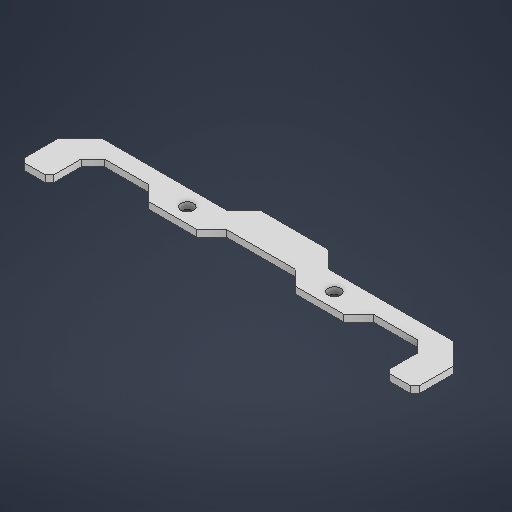
# Autodesk Inventor part: PCBDummy - SenRigFront
Saved by Autodesk Inventor 2027 (Build 310192000, 192)
## iProperties
Created: 2026-09-26
Part Number: PCBDummy - SenRigFront
Material: Všeobecné
Document SubType Name: Modeling
Designer: Vadim
Density: 1 g/cm^3
Appearance: Výchozí
Author: Vadim
Autodesk Inventor part; units mm, degrees
ref_plane "YZ Plane" through (0, 0, 0) normal (1, 0, 0) x (0, 1, 0)
ref_plane "XZ Plane" through (0, 0, 0) normal (0, 1, 0) x (-1, 0, 0)
ref_plane "XY Plane" through (0, 0, 0) normal (0, 0, 1) x (1, 0, 0)
sketch "Náčrt1" plane through (0, 0, 0) normal (0, 1, 0) x (-1, 0, 0)
  line L0 (0, 0) -> (0, -9)
  line L1 (39.5, 0) -> (39.5, 9.8)
  line L2 (39.5, 9.8) -> (47.5, 9.8)
  line L3 (47.5, 9.8) -> (47.5, 0)
  line L4 (47.5, 0) -> (42.5, -5)
  line L5 (42.5, -5) -> (12, -5)
  line L6 (39.5, 0) -> (26.5, 0)
  line L7 (26.5, 0) -> (23.5, 3)
  line L8 (23.5, 3) -> (11.5, 3)
  line L9 (11.5, 3) -> (8.5, 0)
  line L10 (8.5, 0) -> (0, 0)
  circle A0 centre (17.5, -1) radius 1.5
  line L11 (12, -5) -> (8, -9)
  line L12 (8, -9) -> (0, -9)
  line L13 (17.5, 3) -> (17.5, -5) construction
  line L14 (39.5, 2) -> (37.5, 0)
  line L15 (11.7071, 2.5) -> (23.2929, 2.5)
  line L16 (23.2929, 2.5) -> (26.2929, -0.5)
  line L17 (26.2929, -0.5) -> (40, -0.5)
  line L18 (40, -0.5) -> (40, 9.3)
  line L19 (40, 9.3) -> (47, 9.3)
  line L20 (47, 9.3) -> (47, 0.2071)
  line L21 (47, 0.2071) -> (42.2929, -4.5)
  line L22 (42.2929, -4.5) -> (11.7929, -4.5)
  line L23 (11.7929, -4.5) -> (7.7929, -8.5)
  line L24 (7.7929, -8.5) -> (0.5, -8.5)
  line L25 (0.5, -8.5) -> (0.5, -0.5)
  line L26 (0.5, -0.5) -> (8.7071, -0.5)
  line L27 (8.7071, -0.5) -> (11.7071, 2.5)
  line L28 (40, 1.7929) -> (37.7071, -0.5)
  line L29 (0.5, -0.5) -> (0, -0.5)
  line L30 (42.2929, -4.5) -> (41.7929, -5)
  line L31 (37.7071, -0.5) -> (37.2071, -1)
  line L32 (26.7929, -1) -> (26.2929, -0.5)
  line L33 (37.2071, -1) -> (26.7929, -1)
  line L34 (8.7071, -0.5) -> (8.2071, -1)
  line L35 (8.2071, -1) -> (0, -1)
  point P0 (17.5, -1)
  point P1 (38.5, 1)
  point P2 (47, -0.5)
  point P3 (38.2071, 0)
  point P4 (39.5, 1.2929)
  dimension "d1" = 4
  dimension "d2" = 4
  dimension "d3" = 3
  dimension "d4" = 6
  dimension "d5" = 8
  dimension "d6" = 2
  dimension "d7" = 2
  dimension "d8" = 3
  dimension "d9" = 17.5
  dimension "d10" = 5
  dimension "d11" = 5
  dimension "d12" = 14.8
  dimension "d13" = 22
  dimension "d14" = 8
  dimension "d15" = 4
  dimension "d16" = 45
  dimension "d24" = 0.5
  dimension "d25" = 0.5
  dimension "d27" = 0.5
  constraints: 74 end point, 12 perpendicular, 10 point on line, 6 collinear, 6 parallel, 4 midpoint, 2 vertical, 1 centre point, 1 horizontal, 13 other
  measures "d1" distance from line of L5 A0.centre
  measures "d2" distance from line of L8 A0.centre
  measures "d3" diameter of A0
  measures "d4" horizontal distance of A0.centre L7.end
  measures "d5" distance of L1.end L2.end
  measures "d6" distance of L1.start L14.end
  measures "d7" distance of L14.start L1.start
  measures "d8" horizontal distance of L7.end L6.end
  measures "d9" distance from line of L0 point (17.5, -1)
  measures "d10" horizontal distance of L3.end L4.end
  measures "d11" horizontal distance of L3.end L4.end
  measures "d12" distance between parallel lines of L2 L5
  measures "d13" distance from line of L1 point (17.5, -1)
  measures "d14" distance of L11.end L0.end
  measures "d15" distance between parallel lines of L12 L5
  measures "d16" angle of L5 L11
  measures "d24" distance between parallel lines of L6 L17
  measures "d25" distance from line of point (38.5, 1) L28
  measures "d27" distance between parallel lines of L33 L17
extrude "Vysunutí1" add sketch "Náčrt1" along normal blind 1.6 contours L35 L25 L24 L23 L22 L30 L5 L11 L12 L0 | L35 L34 L27 L15 L16 L32 L33 L31 L17 L18 L19 L20 L21 L22 L23 L24 L25 | L28 L1 L6 | L6 L1 L28 L18 L17
chamfer "Zkosení1" distance 1 angle 45 2 edges at (-40, 0.8, 9.3) (-47, 0.8, 9.3)
mirror "Zrcadlit1" about plane through (0, 0, -1) normal (1, 0, 0)
sketch "Náčrt2" plane through (0, 0, 0) normal (0, -1, 0) x (1, 0, 0)
  circle A0 centre (17.5, -1) radius 1.5 projected
  line L0 (-12, -5) -> (-41.7929, -5) projected
  line L1 (-8, -9) -> (-12, -5) projected
  line L2 (-8, -9) -> (8, -9) projected
  line L3 (8, -9) -> (12, -5) projected
  line L4 (12, -5) -> (41.7929, -5) projected
  circle A1 centre (-17.5, -1) radius 1.5 projected
  line L5 (0, -9) -> (0, 0) construction
  line L6 (12, -9) -> (-12, -9) construction
  line L7 (-12, -9) -> (-12, -1) construction
  line L8 (-12, -1) -> (12, -1) construction
  line L9 (12, -1) -> (12, -9) construction
  line L10 (-40, 1.7929) -> (-37.2071, -1) projected
  line L11 (40, 1.7929) -> (37.2071, -1) projected
  line L12 (-47, 8.3) -> (-46, 9.3) projected
  line L13 (-47, 0.2071) -> (-47, 8.3) projected
  line L14 (-41.7929, -5) -> (-47, 0.2071) projected
  line L15 (41.7929, -5) -> (47, 0.2071) projected
  line L16 (47, 0.2071) -> (47, 8.3) projected
  line L17 (47, 8.3) -> (46, 9.3) projected
  line L18 (46, 9.3) -> (41, 9.3) projected
  line L19 (41, 9.3) -> (40, 8.3) projected
  line L20 (40, 8.3) -> (40, 1.7929) projected
  line L21 (26.7929, -1) -> (23.2929, 2.5) projected
  line L22 (23.2929, 2.5) -> (11.7071, 2.5) projected
  line L23 (11.7071, 2.5) -> (8.2071, -1) projected
  line L24 (-11.7071, 2.5) -> (-8.2071, -1) projected
  line L25 (-23.2929, 2.5) -> (-11.7071, 2.5) projected
  line L26 (-26.7929, -1) -> (-23.2929, 2.5) projected
  line L27 (-40, 8.3) -> (-40, 1.7929) projected
  line L28 (-41, 9.3) -> (-40, 8.3) projected
  line L29 (-46, 9.3) -> (-41, 9.3) projected
  line L30 (37.2071, -1) -> (26.7929, -1) projected
  line L31 (-37.2071, -1) -> (-26.7929, -1) projected
  line L32 (-8.2071, -1) -> (8.2071, -1) projected
  spline S0 degree 2 poles (6.8074, -7.598) (6.8074, -7.4522) (6.9114, -7.1896) (7.0044, -7.0984) knots 0 0 0 1 2 2 2
  spline S1 degree 2 poles (7.0044, -7.0984) (7.121, -6.9836) (7.4365, -6.865) (7.6772, -6.865) knots 0 0 0 1 2 2 2
  line L33 (7.6772, -6.865) -> (7.9306, -6.865)
  line L34 (7.9306, -6.865) -> (7.9306, -6.0263)
  line L35 (7.9306, -6.0263) -> (8.2296, -6.0263)
  line L36 (8.2296, -6.0263) -> (8.2296, -8.2763)
  line L37 (8.2296, -8.2763) -> (7.6644, -8.2763)
  spline S2 degree 2 poles (7.6644, -8.2763) (7.4638, -8.2763) (7.183, -8.2107) (7.0755, -8.1359) knots 0 0 0 1 2 2 2
  spline S3 degree 2 poles (7.0755, -8.1359) (6.9497, -8.0502) (6.8074, -7.7858) (6.8074, -7.598) knots 0 0 0 1 2 2 2
  spline S4 degree 2 poles (7.1192, -7.5889) (7.1192, -7.7056) (7.1995, -7.877) (7.2815, -7.9317) knots 0 0 0 1 2 2 2
  spline S5 degree 2 poles (7.2815, -7.9317) (7.3526, -7.9791) (7.5422, -8.0174) (7.6826, -8.0174) knots 0 0 0 1 2 2 2
  line L38 (7.6826, -8.0174) -> (7.9306, -8.0174)
  line L39 (7.9306, -8.0174) -> (7.9306, -7.1203)
  line L40 (7.9306, -7.1203) -> (7.7264, -7.1203)
  spline S6 degree 2 poles (7.7264, -7.1203) (7.5441, -7.1203) (7.3198, -7.1787) (7.2469, -7.2552) knots 0 0 0 1 2 2 2
  spline S7 degree 2 poles (7.2469, -7.2552) (7.1794, -7.3227) (7.1192, -7.4813) (7.1192, -7.5889) knots 0 0 0 1 2 2 2
  spline S8 degree 2 poles (5.6441, -5.9862) (5.8629, -5.9862) (6.2331, -6.1339) (6.368, -6.2816) knots 0 0 0 1 2 2 2
  spline S9 degree 2 poles (6.368, -6.2816) (6.5029, -6.4274) (6.6506, -6.865) (6.6506, -7.1495) knots 0 0 0 1 2 2 2
  spline S10 degree 2 poles (6.6506, -7.1495) (6.6506, -7.4321) (6.5066, -7.8515) (6.3698, -8.0065) knots 0 0 0 1 2 2 2
  spline S11 degree 2 poles (6.3698, -8.0065) (6.2349, -8.1578) (5.8666, -8.3164) (5.6387, -8.3164) knots 0 0 0 1 2 2 2
  spline S12 degree 2 poles (5.6387, -8.3164) (5.5256, -8.3164) (5.3269, -8.2836) (5.243, -8.2581) knots 0 0 0 1 2 2 2
  spline S13 degree 2 poles (5.243, -8.2581) (5.1701, -8.2344) (5.0187, -8.1669) (4.944, -8.1268) knots 0 0 0 1 2 2 2
  line L41 (4.944, -8.1268) -> (4.944, -7.7658)
  line L42 (4.944, -7.7658) -> (4.9677, -7.7658)
  spline S14 degree 2 poles (4.9677, -7.7658) (5.0078, -7.8022) (5.1318, -7.9043) (5.2211, -7.9536) knots 0 0 0 1 2 2 2
  spline S15 degree 2 poles (5.2211, -7.9536) (5.3068, -8.001) (5.5092, -8.0612) (5.6405, -8.0612) knots 0 0 0 1 2 2 2
  spline S16 degree 2 poles (5.6405, -8.0612) (5.7845, -8.0612) (6.0416, -7.9426) (6.1383, -7.8296) knots 0 0 0 1 2 2 2
  spline S17 degree 2 poles (6.1383, -7.8296) (6.2331, -7.7147) (6.3388, -7.3665) (6.3388, -7.1495) knots 0 0 0 1 2 2 2
  spline S18 degree 2 poles (6.3388, -7.1495) (6.3388, -6.9179) (6.2276, -6.5843) (6.131, -6.4694) knots 0 0 0 1 2 2 2
  spline S19 degree 2 poles (6.131, -6.4694) (6.0362, -6.3582) (5.7827, -6.2451) (5.6405, -6.2451) knots 0 0 0 1 2 2 2
  spline S20 degree 2 poles (5.6405, -6.2451) (5.511, -6.2451) (5.2904, -6.3089) (5.2047, -6.3563) knots 0 0 0 1 2 2 2
  spline S21 degree 2 poles (5.2047, -6.3563) (5.1227, -6.4037) (5.0005, -6.5022) (4.9659, -6.5368) knots 0 0 0 1 2 2 2
  line L43 (4.9659, -6.5368) -> (4.944, -6.5368)
  line L44 (4.944, -6.5368) -> (4.944, -6.1795)
  spline S22 degree 2 poles (4.944, -6.1795) (5.0187, -6.1448) (5.15, -6.081) (5.243, -6.0518) knots 0 0 0 1 2 2 2
  spline S23 degree 2 poles (5.243, -6.0518) (5.3415, -6.019) (5.5092, -5.9862) (5.6441, -5.9862) knots 0 0 0 1 2 2 2
  spline S24 degree 2 poles (3.1389, -6.7174) (3.1389, -6.5496) (3.2665, -6.2925) (3.3723, -6.2086) knots 0 0 0 1 2 2 2
  spline S25 degree 2 poles (3.3723, -6.2086) (3.4999, -6.1102) (3.7898, -6.0263) (4.0196, -6.0263) knots 0 0 0 1 2 2 2
  line L45 (4.0196, -6.0263) -> (4.665, -6.0263)
  line L46 (4.665, -6.0263) -> (4.665, -8.2763)
  line L47 (4.665, -8.2763) -> (4.0688, -8.2763)
  spline S26 degree 2 poles (4.0688, -8.2763) (3.8281, -8.2763) (3.5874, -8.2453) (3.478, -8.1851) knots 0 0 0 1 2 2 2
  spline S27 degree 2 poles (3.478, -8.1851) (3.3559, -8.1213) (3.2446, -7.9116) (3.2446, -7.7694) knots 0 0 0 1 2 2 2
  spline S28 degree 2 poles (3.2446, -7.7694) (3.2446, -7.6108) (3.4124, -7.3592) (3.5601, -7.2881) knots 0 0 0 1 2 2 2
  line L48 (3.5601, -7.2881) -> (3.5601, -7.2771)
  spline S29 degree 2 poles (3.5601, -7.2771) (3.3595, -7.2224) (3.1389, -6.9325) (3.1389, -6.7174) knots 0 0 0 1 2 2 2
  spline S30 degree 2 poles (3.4507, -6.7046) (3.4507, -6.8322) (3.5236, -6.9963) (3.633, -7.0547) knots 0 0 0 1 2 2 2
  spline S31 degree 2 poles (3.633, -7.0547) (3.7041, -7.0911) (3.8719, -7.113) (4.0268, -7.113) knots 0 0 0 1 2 2 2
  line L49 (4.0268, -7.113) -> (4.366, -7.113)
  line L50 (4.366, -7.113) -> (4.366, -6.2816)
  line L51 (4.366, -6.2816) -> (4.1235, -6.2816)
  spline S32 degree 2 poles (4.1235, -6.2816) (3.9266, -6.2816) (3.7005, -6.318) (3.6129, -6.3764) knots 0 0 0 1 2 2 2
  spline S33 degree 2 poles (3.6129, -6.3764) (3.5291, -6.4366) (3.4507, -6.5861) (3.4507, -6.7046) knots 0 0 0 1 2 2 2
  spline S34 degree 2 poles (3.5564, -7.7275) (3.5564, -7.8077) (3.6111, -7.9281) (3.6713, -7.9627) knots 0 0 0 1 2 2 2
  spline S35 degree 2 poles (3.6713, -7.9627) (3.7442, -8.0028) (3.9211, -8.021) (4.0797, -8.021) knots 0 0 0 1 2 2 2
  line L52 (4.0797, -8.021) -> (4.366, -8.021)
  line L53 (4.366, -8.021) -> (4.366, -7.3628)
  line L54 (4.366, -7.3628) -> (4.0268, -7.3628)
  spline S36 degree 2 poles (4.0268, -7.3628) (3.8864, -7.3628) (3.7533, -7.392) (3.6822, -7.4376) knots 0 0 0 1 2 2 2
  spline S37 degree 2 poles (3.6822, -7.4376) (3.6129, -7.4813) (3.5564, -7.6217) (3.5564, -7.7275) knots 0 0 0 1 2 2 2
  spline S38 degree 2 poles (0.1012, -7.1495) (0.1012, -6.8413) (0.351, -6.3454) (0.5607, -6.2068) knots 0 0 0 1 2 2 2
  spline S39 degree 2 poles (0.5607, -6.2068) (0.7321, -6.0992) (1.084, -6.0263) (1.3575, -6.0263) knots 0 0 0 1 2 2 2
  line L55 (1.3575, -6.0263) -> (1.8753, -6.0263)
  line L56 (1.8753, -6.0263) -> (1.8753, -8.2763)
  line L57 (1.8753, -8.2763) -> (1.3629, -8.2763)
  spline S40 degree 2 poles (1.3629, -8.2763) (1.0457, -8.2763) (0.6847, -8.1815) (0.557, -8.0976) knots 0 0 0 1 2 2 2
  spline S41 degree 2 poles (0.557, -8.0976) (0.3401, -7.9536) (0.1012, -7.4777) (0.1012, -7.1495) knots 0 0 0 1 2 2 2
  spline S42 degree 2 poles (0.413, -7.1531) (0.413, -7.412) (0.5844, -7.7785) (0.754, -7.8825) knots 0 0 0 1 2 2 2
  spline S43 degree 2 poles (0.754, -7.8825) (0.8743, -7.9536) (1.146, -8.0174) (1.3484, -8.0174) knots 0 0 0 1 2 2 2
  line L58 (1.3484, -8.0174) -> (1.5763, -8.0174)
  line L59 (1.5763, -8.0174) -> (1.5763, -6.2852)
  line L60 (1.5763, -6.2852) -> (1.3484, -6.2852)
  spline S44 degree 2 poles (1.3484, -6.2852) (1.1496, -6.2852) (0.8488, -6.349) (0.7266, -6.4347) knots 0 0 0 1 2 2 2
  spline S45 degree 2 poles (0.7266, -6.4347) (0.5698, -6.5405) (0.413, -6.8906) (0.413, -7.1531) knots 0 0 0 1 2 2 2
  line L61 (-1.5143, -6.0263) -> (-1.2298, -6.0263)
  line L62 (-1.2298, -6.0263) -> (-1.2298, -6.2123)
  spline S46 degree 2 poles (-1.2298, -6.2123) (-1.0986, -6.0974) (-0.8634, -5.9789) (-0.7175, -5.9789) knots 0 0 0 1 2 2 2
  spline S47 degree 2 poles (-0.7175, -5.9789) (-0.6081, -5.9789) (-0.413, -6.0518) (-0.3419, -6.1302) knots 0 0 0 1 2 2 2
  spline S48 degree 2 poles (-0.3419, -6.1302) (-0.2689, -6.2086) (-0.1887, -6.4475) (-0.1887, -6.6189) knots 0 0 0 1 2 2 2
  line L63 (-0.1887, -6.6189) -> (-0.1887, -7.7147)
  line L64 (-0.1887, -7.7147) -> (-0.4732, -7.7147)
  line L65 (-0.4732, -7.7147) -> (-0.4732, -6.752)
  spline S49 degree 2 poles (-0.4732, -6.752) (-0.4732, -6.6171) (-0.4932, -6.4402) (-0.5279, -6.3746) knots 0 0 0 1 2 2 2
  spline S50 degree 2 poles (-0.5279, -6.3746) (-0.5625, -6.3089) (-0.681, -6.2488) (-0.7922, -6.2488) knots 0 0 0 1 2 2 2
  spline S51 degree 2 poles (-0.7922, -6.2488) (-0.8962, -6.2488) (-1.1314, -6.3673) (-1.2298, -6.453) knots 0 0 0 1 2 2 2
  line L66 (-1.2298, -6.453) -> (-1.2298, -7.7147)
  line L67 (-1.2298, -7.7147) -> (-1.5143, -7.7147)
  line L68 (-1.5143, -7.7147) -> (-1.5143, -6.0263)
  line L69 (-3.8409, -6.0263) -> (-3.8409, -7.0036)
  spline S52 degree 2 poles (-3.8409, -7.0036) (-3.8409, -7.1203) (-3.8226, -7.3191) (-3.7935, -7.3738) knots 0 0 0 1 2 2 2
  spline S53 degree 2 poles (-3.7935, -7.3738) (-3.7643, -7.4339) (-3.6531, -7.4923) (-3.5564, -7.4923) knots 0 0 0 1 2 2 2
  spline S54 degree 2 poles (-3.5564, -7.4923) (-3.4689, -7.4923) (-3.2683, -7.3847) (-3.1626, -7.2826) knots 0 0 0 1 2 2 2
  spline S55 degree 2 poles (-3.1626, -7.2826) (-3.1644, -7.2571) (-3.1681, -7.186) (-3.1681, -7.1385) knots 0 0 0 1 2 2 2
  line L70 (-3.1681, -7.1385) -> (-3.1681, -6.0263)
  line L71 (-3.1681, -6.0263) -> (-2.8836, -6.0263)
  line L72 (-2.8836, -6.0263) -> (-2.8836, -7.0036)
  spline S56 degree 2 poles (-2.8836, -7.0036) (-2.8836, -7.1203) (-2.8654, -7.3191) (-2.8362, -7.3738) knots 0 0 0 1 2 2 2
  spline S57 degree 2 poles (-2.8362, -7.3738) (-2.807, -7.4339) (-2.6958, -7.4923) (-2.5992, -7.4923) knots 0 0 0 1 2 2 2
  spline S58 degree 2 poles (-2.5992, -7.4923) (-2.508, -7.4923) (-2.3056, -7.3774) (-2.2108, -7.2881) knots 0 0 0 1 2 2 2
  line L73 (-2.2108, -7.2881) -> (-2.2108, -6.0263)
  line L74 (-2.2108, -6.0263) -> (-1.9264, -6.0263)
  line L75 (-1.9264, -6.0263) -> (-1.9264, -7.7147)
  line L76 (-1.9264, -7.7147) -> (-2.2108, -7.7147)
  line L77 (-2.2108, -7.7147) -> (-2.2108, -7.5287)
  spline S59 degree 2 poles (-2.2108, -7.5287) (-2.322, -7.64) (-2.5408, -7.7621) (-2.6721, -7.7621) knots 0 0 0 1 2 2 2
  spline S60 degree 2 poles (-2.6721, -7.7621) (-2.8216, -7.7621) (-3.0532, -7.6254) (-3.1134, -7.4704) knots 0 0 0 1 2 2 2
  spline S61 degree 2 poles (-3.1134, -7.4704) (-3.2428, -7.6144) (-3.4871, -7.7621) (-3.6294, -7.7621) knots 0 0 0 1 2 2 2
  spline S62 degree 2 poles (-3.6294, -7.7621) (-3.7388, -7.7621) (-3.9174, -7.6947) (-3.9831, -7.6181) knots 0 0 0 1 2 2 2
  spline S63 degree 2 poles (-3.9831, -7.6181) (-4.0505, -7.5415) (-4.1253, -7.3118) (-4.1253, -7.1385) knots 0 0 0 1 2 2 2
  line L78 (-4.1253, -7.1385) -> (-4.1253, -6.0263)
  line L79 (-4.1253, -6.0263) -> (-3.8409, -6.0263)
  line L80 (-6.4391, -6.0263) -> (-6.4391, -7.0036)
  spline S64 degree 2 poles (-6.4391, -7.0036) (-6.4391, -7.1203) (-6.4209, -7.3191) (-6.3917, -7.3738) knots 0 0 0 1 2 2 2
  spline S65 degree 2 poles (-6.3917, -7.3738) (-6.3625, -7.4339) (-6.2513, -7.4923) (-6.1547, -7.4923) knots 0 0 0 1 2 2 2
  spline S66 degree 2 poles (-6.1547, -7.4923) (-6.0672, -7.4923) (-5.8666, -7.3847) (-5.7608, -7.2826) knots 0 0 0 1 2 2 2
  spline S67 degree 2 poles (-5.7608, -7.2826) (-5.7627, -7.2571) (-5.7663, -7.186) (-5.7663, -7.1385) knots 0 0 0 1 2 2 2
  line L81 (-5.7663, -7.1385) -> (-5.7663, -6.0263)
  line L82 (-5.7663, -6.0263) -> (-5.4819, -6.0263)
  line L83 (-5.4819, -6.0263) -> (-5.4819, -7.0036)
  spline S68 degree 2 poles (-5.4819, -7.0036) (-5.4819, -7.1203) (-5.4636, -7.3191) (-5.4345, -7.3738) knots 0 0 0 1 2 2 2
  spline S69 degree 2 poles (-5.4345, -7.3738) (-5.4053, -7.4339) (-5.2941, -7.4923) (-5.1974, -7.4923) knots 0 0 0 1 2 2 2
  spline S70 degree 2 poles (-5.1974, -7.4923) (-5.1063, -7.4923) (-4.9039, -7.3774) (-4.8091, -7.2881) knots 0 0 0 1 2 2 2
  line L84 (-4.8091, -7.2881) -> (-4.8091, -6.0263)
  line L85 (-4.8091, -6.0263) -> (-4.5246, -6.0263)
  line L86 (-4.5246, -6.0263) -> (-4.5246, -7.7147)
  line L87 (-4.5246, -7.7147) -> (-4.8091, -7.7147)
  line L88 (-4.8091, -7.7147) -> (-4.8091, -7.5287)
  spline S71 degree 2 poles (-4.8091, -7.5287) (-4.9203, -7.64) (-5.1391, -7.7621) (-5.2704, -7.7621) knots 0 0 0 1 2 2 2
  spline S72 degree 2 poles (-5.2704, -7.7621) (-5.4199, -7.7621) (-5.6514, -7.6254) (-5.7116, -7.4704) knots 0 0 0 1 2 2 2
  spline S73 degree 2 poles (-5.7116, -7.4704) (-5.8411, -7.6144) (-6.0854, -7.7621) (-6.2276, -7.7621) knots 0 0 0 1 2 2 2
  spline S74 degree 2 poles (-6.2276, -7.7621) (-6.337, -7.7621) (-6.5157, -7.6947) (-6.5813, -7.6181) knots 0 0 0 1 2 2 2
  spline S75 degree 2 poles (-6.5813, -7.6181) (-6.6488, -7.5415) (-6.7236, -7.3118) (-6.7236, -7.1385) knots 0 0 0 1 2 2 2
  line L89 (-6.7236, -7.1385) -> (-6.7236, -6.0263)
  line L90 (-6.7236, -6.0263) -> (-6.4391, -6.0263)
  line L91 (-8.4484, -7.7147) -> (-7.5404, -5.4046)
  line L92 (-7.5404, -5.4046) -> (-7.2359, -5.4046)
  line L93 (-7.2359, -5.4046) -> (-7.5386, -6.1084)
  line L94 (-7.5386, -6.1084) -> (-6.926, -7.7147)
  line L95 (-6.926, -7.7147) -> (-7.2323, -7.7147)
  line L96 (-7.2323, -7.7147) -> (-7.6936, -6.4639)
  line L97 (-7.6936, -6.4639) -> (-8.1531, -7.7147)
  line L98 (-8.1531, -7.7147) -> (-8.4484, -7.7147)
  spline S76 degree 2 poles (7.4365, -2.2816) (7.6808, -2.2816) (8.0236, -2.3837) (8.1749, -2.4567) knots 0 0 0 1 2 2 2
  line L99 (8.1749, -2.4567) -> (8.1749, -2.8323)
  line L100 (8.1749, -2.8323) -> (8.1531, -2.8323)
  spline S77 degree 2 poles (8.1531, -2.8323) (8.0054, -2.6937) (7.6316, -2.5405) (7.4584, -2.5405) knots 0 0 0 1 2 2 2
  spline S78 degree 2 poles (7.4584, -2.5405) (7.2104, -2.5405) (6.9569, -2.7466) (6.9569, -2.9162) knots 0 0 0 1 2 2 2
  spline S79 degree 2 poles (6.9569, -2.9162) (6.9569, -3.0511) (7.0901, -3.2188) (7.2341, -3.2608) knots 0 0 0 1 2 2 2
  spline S80 degree 2 poles (7.2341, -3.2608) (7.338, -3.2899) (7.5112, -3.3301) (7.6407, -3.3629) knots 0 0 0 1 2 2 2
  spline S81 degree 2 poles (7.6407, -3.3629) (7.7574, -3.3939) (7.9416, -3.4869) (8.0127, -3.5616) knots 0 0 0 1 2 2 2
  spline S82 degree 2 poles (8.0127, -3.5616) (8.0819, -3.6364) (8.1585, -3.8369) (8.1585, -3.9682) knots 0 0 0 1 2 2 2
  spline S83 degree 2 poles (8.1585, -3.9682) (8.1585, -4.2417) (7.7319, -4.6119) (7.4018, -4.6119) knots 0 0 0 1 2 2 2
  spline S84 degree 2 poles (7.4018, -4.6119) (7.2122, -4.6119) (6.8767, -4.5371) (6.7327, -4.466) knots 0 0 0 1 2 2 2
  line L101 (6.7327, -4.466) -> (6.7327, -4.1086)
  line L102 (6.7327, -4.1086) -> (6.7546, -4.1086)
  spline S85 degree 2 poles (6.7546, -4.1086) (6.8621, -4.2071) (7.1976, -4.3529) (7.3818, -4.3529) knots 0 0 0 1 2 2 2
  spline S86 degree 2 poles (7.3818, -4.3529) (7.5896, -4.3529) (7.8467, -4.1578) (7.8467, -3.9992) knots 0 0 0 1 2 2 2
  spline S87 degree 2 poles (7.8467, -3.9992) (7.8467, -3.857) (7.6954, -3.6874) (7.5532, -3.6491) knots 0 0 0 1 2 2 2
  spline S88 degree 2 poles (7.5532, -3.6491) (7.4584, -3.6236) (7.183, -3.558) (7.0919, -3.5306) knots 0 0 0 1 2 2 2
  spline S89 degree 2 poles (7.0919, -3.5306) (6.8603, -3.4595) (6.6452, -3.1732) (6.6452, -2.9636) knots 0 0 0 1 2 2 2
  spline S90 degree 2 poles (6.6452, -2.9636) (6.6452, -2.8305) (6.7527, -2.5752) (6.8494, -2.4858) knots 0 0 0 1 2 2 2
  spline S91 degree 2 poles (6.8494, -2.4858) (6.9569, -2.3874) (7.2304, -2.2816) (7.4365, -2.2816) knots 0 0 0 1 2 2 2
  spline S92 degree 2 poles (5.6296, -2.2835) (6.0343, -2.2835) (6.4792, -2.7375) (6.4792, -3.1568) knots 0 0 0 1 2 2 2
  spline S93 degree 2 poles (6.4792, -3.1568) (6.4792, -3.5689) (6.0471, -4.0576) (5.6988, -4.0576) knots 0 0 0 1 2 2 2
  spline S94 degree 2 poles (5.6988, -4.0576) (5.542, -4.0576) (5.2995, -3.9664) (5.2102, -3.8698) knots 0 0 0 1 2 2 2
  spline S95 degree 2 poles (5.2102, -3.8698) (5.119, -3.7731) (5.0224, -3.4942) (5.0224, -3.2918) knots 0 0 0 1 2 2 2
  line L103 (5.0224, -3.2918) -> (5.0224, -3.1368)
  line L104 (5.0224, -3.1368) -> (6.1911, -3.1368)
  spline S96 degree 2 poles (6.1911, -3.1368) (6.1911, -2.8432) (5.8958, -2.5314) (5.6332, -2.5314) knots 0 0 0 1 2 2 2
  spline S97 degree 2 poles (5.6332, -2.5314) (5.5402, -2.5314) (5.3597, -2.5734) (5.2868, -2.6062) knots 0 0 0 1 2 2 2
  spline S98 degree 2 poles (5.2868, -2.6062) (5.2102, -2.6427) (5.1044, -2.7065) (5.0698, -2.7356) knots 0 0 0 1 2 2 2
  line L105 (5.0698, -2.7356) -> (5.0534, -2.7356)
  line L106 (5.0534, -2.7356) -> (5.0534, -2.4257)
  spline S99 degree 2 poles (5.0534, -2.4257) (5.1026, -2.4056) (5.2521, -2.3473) (5.3105, -2.3309) knots 0 0 0 1 2 2 2
  spline S100 degree 2 poles (5.3105, -2.3309) (5.3925, -2.3072) (5.5275, -2.2835) (5.6296, -2.2835) knots 0 0 0 1 2 2 2
  spline S101 degree 2 poles (5.2995, -3.3538) (5.3032, -3.4686) (5.3506, -3.6364) (5.3962, -3.6929) knots 0 0 0 1 2 2 2
  spline S102 degree 2 poles (5.3962, -3.6929) (5.4454, -3.7567) (5.6004, -3.8242) (5.7153, -3.8242) knots 0 0 0 1 2 2 2
  spline S103 degree 2 poles (5.7153, -3.8242) (5.8283, -3.8242) (5.9869, -3.7567) (6.0526, -3.6911) knots 0 0 0 1 2 2 2
  spline S104 degree 2 poles (6.0526, -3.6911) (6.1164, -3.6236) (6.182, -3.4613) (6.1911, -3.3538) knots 0 0 0 1 2 2 2
  line L107 (6.1911, -3.3538) -> (5.2995, -3.3538)
  line L108 (3.4087, -2.3217) -> (3.6932, -2.3217)
  line L109 (3.6932, -2.3217) -> (3.6932, -3.2845)
  spline S105 degree 2 poles (3.6932, -3.2845) (3.6932, -3.4012) (3.7151, -3.6017) (3.7479, -3.6619) knots 0 0 0 1 2 2 2
  spline S106 degree 2 poles (3.7479, -3.6619) (3.7825, -3.7257) (3.9065, -3.7877) (4.0123, -3.7877) knots 0 0 0 1 2 2 2
  spline S107 degree 2 poles (4.0123, -3.7877) (4.118, -3.7877) (4.3423, -3.6747) (4.4499, -3.5835) knots 0 0 0 1 2 2 2
  line L110 (4.4499, -3.5835) -> (4.4499, -2.3217)
  line L111 (4.4499, -2.3217) -> (4.7343, -2.3217)
  line L112 (4.7343, -2.3217) -> (4.7343, -4.0102)
  line L113 (4.7343, -4.0102) -> (4.4499, -4.0102)
  line L114 (4.4499, -4.0102) -> (4.4499, -3.8224)
  spline S108 degree 2 poles (4.4499, -3.8224) (4.3222, -3.9372) (4.0761, -4.0576) (3.9375, -4.0576) knots 0 0 0 1 2 2 2
  spline S109 degree 2 poles (3.9375, -4.0576) (3.6895, -4.0576) (3.4087, -3.7294) (3.4087, -3.4176) knots 0 0 0 1 2 2 2
  line L115 (3.4087, -3.4176) -> (3.4087, -2.3217)
  line L116 (1.2463, -2.3217) -> (1.6346, -2.3217)
  line L117 (1.6346, -2.3217) -> (2.3457, -3.217)
  line L118 (2.3457, -3.217) -> (2.6885, -3.217)
  line L119 (2.6885, -3.217) -> (2.6885, -2.3217)
  line L120 (2.6885, -2.3217) -> (2.9875, -2.3217)
  line L121 (2.9875, -2.3217) -> (2.9875, -4.5717)
  line L122 (2.9875, -4.5717) -> (2.4077, -4.5717)
  spline S110 degree 2 poles (2.4077, -4.5717) (2.2144, -4.5717) (1.9537, -4.5298) (1.8352, -4.4532) knots 0 0 0 1 2 2 2
  spline S111 degree 2 poles (1.8352, -4.4532) (1.7167, -4.3766) (1.5799, -4.1378) (1.5799, -3.9609) knots 0 0 0 1 2 2 2
  spline S112 degree 2 poles (1.5799, -3.9609) (1.5799, -3.7148) (1.8315, -3.3811) (2.0467, -3.3009) knots 0 0 0 1 2 2 2
  line L123 (2.0467, -3.3009) -> (1.2463, -2.3217)
  spline S113 degree 2 poles (1.8917, -3.9372) (1.8917, -4.0357) (1.961, -4.187) (2.0339, -4.2363) knots 0 0 0 1 2 2 2
  spline S114 degree 2 poles (2.0339, -4.2363) (2.0978, -4.2782) (2.2673, -4.3128) (2.3913, -4.3128) knots 0 0 0 1 2 2 2
  line L124 (2.3913, -4.3128) -> (2.6885, -4.3128)
  line L125 (2.6885, -4.3128) -> (2.6885, -3.4668)
  line L126 (2.6885, -3.4668) -> (2.426, -3.4668)
  spline S115 degree 2 poles (2.426, -3.4668) (2.2965, -3.4668) (2.0905, -3.5124) (2.0193, -3.5835) knots 0 0 0 1 2 2 2
  spline S116 degree 2 poles (2.0193, -3.5835) (1.9537, -3.6455) (1.8917, -3.8205) (1.8917, -3.9372) knots 0 0 0 1 2 2 2
  line L127 (0.7995, -2.3217) -> (1.084, -2.3217)
  line L128 (1.084, -2.3217) -> (1.084, -4.0102)
  line L129 (1.084, -4.0102) -> (0.7995, -4.0102)
  line L130 (0.7995, -4.0102) -> (0.7995, -2.3217)
  line L131 (0.7795, -4.291) -> (1.1022, -4.291)
  line L132 (1.1022, -4.291) -> (1.1022, -4.5863)
  line L133 (1.1022, -4.5863) -> (0.7795, -4.5863)
  line L134 (0.7795, -4.5863) -> (0.7795, -4.291)
  spline S117 degree 2 poles (0.3218, -2.0519) (0.2926, -2.0391) (0.1814, -1.999) (0.1103, -1.9826) knots 0 0 0 1 2 2 2
  spline S118 degree 2 poles (0.1103, -1.9826) (0.0319, -1.9625) (-0.1012, -1.9388) (-0.1796, -1.9388) knots 0 0 0 1 2 2 2
  spline S119 degree 2 poles (-0.1796, -1.9388) (-0.3109, -1.9388) (-0.4932, -2.0081) (-0.5443, -2.0701) knots 0 0 0 1 2 2 2
  spline S120 degree 2 poles (-0.5443, -2.0701) (-0.5935, -2.1321) (-0.6318, -2.2944) (-0.6318, -2.3983) knots 0 0 0 1 2 2 2
  line L135 (-0.6318, -2.3983) -> (-0.6318, -2.546)
  spline S121 degree 2 poles (-0.6318, -2.546) (-0.5169, -2.4457) (-0.2963, -2.3509) (-0.1304, -2.3509) knots 0 0 0 1 2 2 2
  spline S122 degree 2 poles (-0.1304, -2.3509) (0.1577, -2.3509) (0.4987, -2.7794) (0.4987, -3.1824) knots 0 0 0 1 2 2 2
  spline S123 degree 2 poles (0.4987, -3.1824) (0.4987, -3.392) (0.3802, -3.7166) (0.2817, -3.8315) knots 0 0 0 1 2 2 2
  spline S124 degree 2 poles (0.2817, -3.8315) (0.1869, -3.939) (-0.0738, -4.0576) (-0.2124, -4.0576) knots 0 0 0 1 2 2 2
  spline S125 degree 2 poles (-0.2124, -4.0576) (-0.3437, -4.0576) (-0.5352, -3.9956) (-0.6318, -3.939) knots 0 0 0 1 2 2 2
  line L136 (-0.6318, -3.939) -> (-0.6482, -4.0102)
  line L137 (-0.6482, -4.0102) -> (-0.9162, -4.0102)
  line L138 (-0.9162, -4.0102) -> (-0.9162, -2.515)
  spline S126 degree 2 poles (-0.9162, -2.515) (-0.9162, -2.0847) (-0.5424, -1.6836) (-0.1577, -1.6836) knots 0 0 0 1 2 2 2
  spline S127 degree 2 poles (-0.1577, -1.6836) (-0.0337, -1.6836) (0.2252, -1.7237) (0.3364, -1.7565) knots 0 0 0 1 2 2 2
  line L139 (0.3364, -1.7565) -> (0.3364, -2.0519)
  line L140 (0.3364, -2.0519) -> (0.3218, -2.0519)
  line L141 (-0.6318, -2.7794) -> (-0.6318, -3.7075)
  spline S128 degree 2 poles (-0.6318, -3.7075) (-0.526, -3.7585) (-0.3473, -3.8023) (-0.258, -3.8023) knots 0 0 0 1 2 2 2
  spline S129 degree 2 poles (-0.258, -3.8023) (-0.0428, -3.8023) (0.2051, -3.485) (0.2051, -3.1878) knots 0 0 0 1 2 2 2
  spline S130 degree 2 poles (0.2051, -3.1878) (0.2051, -2.907) (0.0173, -2.6135) (-0.1942, -2.6135) knots 0 0 0 1 2 2 2
  spline S131 degree 2 poles (-0.1942, -2.6135) (-0.3054, -2.6135) (-0.5388, -2.701) (-0.6318, -2.7794) knots 0 0 0 1 2 2 2
  line L142 (-2.6958, -4.3055) -> (-1.6492, -4.3055)
  line L143 (-1.6492, -4.3055) -> (-1.6492, -3.671)
  line L144 (-1.6492, -3.671) -> (-2.652, -3.671)
  line L145 (-2.652, -3.671) -> (-2.652, -3.4048)
  line L146 (-2.652, -3.4048) -> (-1.6492, -3.4048)
  line L147 (-1.6492, -3.4048) -> (-1.6492, -2.3217)
  line L148 (-1.6492, -2.3217) -> (-1.3502, -2.3217)
  line L149 (-1.3502, -2.3217) -> (-1.3502, -4.5717)
  line L150 (-1.3502, -4.5717) -> (-2.6958, -4.5717)
  line L151 (-2.6958, -4.5717) -> (-2.6958, -4.3055)
  line L152 (-3.8372, -3.7057) -> (-3.8226, -3.7057)
  spline S132 degree 2 poles (-3.8226, -3.7057) (-3.7898, -3.7148) (-3.7187, -3.7184) (-3.6695, -3.7184) knots 0 0 0 1 2 2 2
  spline S133 degree 2 poles (-3.6695, -3.7184) (-3.5546, -3.7184) (-3.3285, -3.6181) (-3.2264, -3.5197) knots 0 0 0 1 2 2 2
  line L153 (-3.2264, -3.5197) -> (-3.2264, -2.3217)
  line L154 (-3.2264, -2.3217) -> (-2.942, -2.3217)
  line L155 (-2.942, -2.3217) -> (-2.942, -4.0102)
  line L156 (-2.942, -4.0102) -> (-3.2264, -4.0102)
  line L157 (-3.2264, -4.0102) -> (-3.2264, -3.7585)
  spline S134 degree 2 poles (-3.2264, -3.7585) (-3.3814, -3.8971) (-3.6129, -4.0102) (-3.7223, -4.0102) knots 0 0 0 1 2 2 2
  spline S135 degree 2 poles (-3.7223, -4.0102) (-3.7661, -4.0102) (-3.8099, -4.0065) (-3.8372, -4.001) knots 0 0 0 1 2 2 2
  line L158 (-3.8372, -4.001) -> (-3.8372, -3.7057)
  spline S136 degree 2 poles (-5.4454, -3.166) (-5.4454, -2.7393) (-5.0351, -2.2743) (-4.6924, -2.2743) knots 0 0 0 1 2 2 2
  spline S137 degree 2 poles (-4.6924, -2.2743) (-4.3405, -2.2743) (-3.9375, -2.7539) (-3.9375, -3.166) knots 0 0 0 1 2 2 2
  spline S138 degree 2 poles (-3.9375, -3.166) (-3.9375, -3.589) (-4.3532, -4.0576) (-4.6924, -4.0576) knots 0 0 0 1 2 2 2
  spline S139 degree 2 poles (-4.6924, -4.0576) (-5.0351, -4.0576) (-5.4454, -3.5908) (-5.4454, -3.166) knots 0 0 0 1 2 2 2
  spline S140 degree 2 poles (-5.1518, -3.166) (-5.1518, -3.4942) (-4.913, -3.8132) (-4.6924, -3.8132) knots 0 0 0 1 2 2 2
  spline S141 degree 2 poles (-4.6924, -3.8132) (-4.4717, -3.8132) (-4.2311, -3.4942) (-4.2311, -3.166) knots 0 0 0 1 2 2 2
  spline S142 degree 2 poles (-4.2311, -3.166) (-4.2311, -2.8469) (-4.4717, -2.5187) (-4.6924, -2.5187) knots 0 0 0 1 2 2 2
  spline S143 degree 2 poles (-4.6924, -2.5187) (-4.9112, -2.5187) (-5.1518, -2.8414) (-5.1518, -3.166) knots 0 0 0 1 2 2 2
  line L159 (-7.0627, -2.3217) -> (-6.7783, -2.3217)
  line L160 (-6.7783, -2.3217) -> (-6.7783, -3.2845)
  spline S144 degree 2 poles (-6.7783, -3.2845) (-6.7783, -3.4012) (-6.7564, -3.6017) (-6.7236, -3.6619) knots 0 0 0 1 2 2 2
  spline S145 degree 2 poles (-6.7236, -3.6619) (-6.6889, -3.7257) (-6.5649, -3.7877) (-6.4592, -3.7877) knots 0 0 0 1 2 2 2
  spline S146 degree 2 poles (-6.4592, -3.7877) (-6.3534, -3.7877) (-6.1292, -3.6747) (-6.0216, -3.5835) knots 0 0 0 1 2 2 2
  line L161 (-6.0216, -3.5835) -> (-6.0216, -2.3217)
  line L162 (-6.0216, -2.3217) -> (-5.7371, -2.3217)
  line L163 (-5.7371, -2.3217) -> (-5.7371, -4.0102)
  line L164 (-5.7371, -4.0102) -> (-6.0216, -4.0102)
  line L165 (-6.0216, -4.0102) -> (-6.0216, -3.8224)
  spline S147 degree 2 poles (-6.0216, -3.8224) (-6.1492, -3.9372) (-6.3954, -4.0576) (-6.5339, -4.0576) knots 0 0 0 1 2 2 2
  spline S148 degree 2 poles (-6.5339, -4.0576) (-6.7819, -4.0576) (-7.0627, -3.7294) (-7.0627, -3.4176) knots 0 0 0 1 2 2 2
  line L166 (-7.0627, -3.4176) -> (-7.0627, -2.3217)
  spline S149 degree 2 poles (-7.9725, -2.2889) (-7.741, -2.2889) (-7.4802, -2.5533) (-7.4802, -2.8396) knots 0 0 0 1 2 2 2
  line L167 (-7.4802, -2.8396) -> (-7.4802, -3.7749)
  line L168 (-7.4802, -3.7749) -> (-7.2888, -3.7749)
  line L169 (-7.2888, -3.7749) -> (-7.2888, -4.0102)
  line L170 (-7.2888, -4.0102) -> (-7.4802, -4.0102)
  line L171 (-7.4802, -4.0102) -> (-7.4802, -4.4952)
  line L172 (-7.4802, -4.4952) -> (-7.7647, -4.4952)
  line L173 (-7.7647, -4.4952) -> (-7.7647, -4.0102)
  line L174 (-7.7647, -4.0102) -> (-8.288, -4.0102)
  line L175 (-8.288, -4.0102) -> (-8.288, -3.7749)
  line L176 (-8.288, -3.7749) -> (-7.7647, -3.7749)
  line L177 (-7.7647, -3.7749) -> (-7.7647, -2.9709)
  spline S150 degree 2 poles (-7.7647, -2.9709) (-7.7647, -2.8432) (-7.7738, -2.7028) (-7.8048, -2.6427) knots 0 0 0 1 2 2 2
  spline S151 degree 2 poles (-7.8048, -2.6427) (-7.8303, -2.5898) (-7.9452, -2.5369) (-8.0437, -2.5369) knots 0 0 0 1 2 2 2
  spline S152 degree 2 poles (-8.0437, -2.5369) (-8.1129, -2.5369) (-8.2424, -2.5788) (-8.2716, -2.5916) knots 0 0 0 1 2 2 2
  line L178 (-8.2716, -2.5916) -> (-8.288, -2.5916)
  line L179 (-8.288, -2.5916) -> (-8.288, -2.3363)
  spline S153 degree 2 poles (-8.288, -2.3363) (-8.2078, -2.3145) (-8.0437, -2.2889) (-7.9725, -2.2889) knots 0 0 0 1 2 2 2
  constraints: 3 midpoint, 2 collinear, 2 end point, 1 vertical, 2 other
extrude "Vysunutí2" cut sketch "Náčrt2" against normal blind 0.2 contours S0 S1 L33 L34 L35 L36 L37 S2 S3 | S8 S9 S10 S11 S12 S13 L41 L42 S14 S15 S16 S17 S18 S19 S20 S21 L43 L44 S22 S23 | S24 S25 L45 L46 L47 S26 S27 S28 L48 S29 | S38 S39 L55 L56 L57 S40 S41 | L61 L62 S46 S47 S48 L63 L64 L65 S49 S50 S51 L66 L67 L68 | L69 S52 S53 S54 S55 L70 L71 L72 S56 S57 S58 L73 L74 L75 L76 L77 S59 S60 S61 S62 S63 L78 L79 | L80 S64 S65 S66 S67 L81 L82 L83 S68 S69 S70 L84 L85 L86 L87 L88 S71 S72 S73 S74 S75 L89 L90 | L91 L92 L93 L94 L95 L96 L97 L98 | S76 L99 L100 S77 S78 S79 S80 S81 S82 S83 S84 L101 L102 S85 S86 S87 S88 S89 S90 S91 | S92 S93 S94 S95 L103 L104 S96 S97 S98 L105 L106 S99 S100 | L108 L109 S105 S106 S107 L110 L111 L112 L113 L114 S108 S109 L115 | L116 L117 L118 L119 L120 L121 L122 S110 S111 S112 L123 | L127 L128 L129 L130 | L131 L132 L133 L134 | S117 S118 S119 S120 L135 S121 S122 S123 S124 S125 L136 L137 L138 S126 S127 L139 L140 | L142 L143 L144 L145 L146 L147 L148 L149 L150 L151 | L152 S132 S133 L153 L154 L155 L156 L157 S134 S135 L158 | S136 S137 S138 S139 | L159 L160 S144 S145 S146 L161 L162 L163 L164 L165 S147 S148 L166 | S149 L167 L168 L169 L170 L171 L172 L173 L174 L175 L176 L177 S150 S151 S152 L178 L179 S153
equation "\"d7\" = d6"
equation "\"d11\" = d10"
equation "\"d25\" = d24"
equation "\"d27\" = d24"
